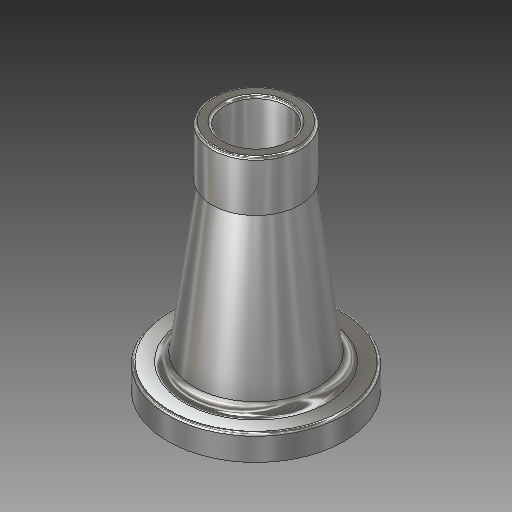
# Autodesk Inventor part: Body
Saved by Autodesk Inventor 2018 (Build 220112000, 112)
## iProperties
Created: 2019-08-24
Part Number: Body
Material: Generic
Document SubType Name: Modeling
Designer: HP
Density: 1 g/cm^3
Appearance: Chrome - Polished
Author: HP
Autodesk Inventor part; units mm, degrees
ref_plane "YZ Plane" through (0, 0, 0) normal (1, 0, 0) x (0, 1, 0)
ref_plane "XZ Plane" through (0, 0, 0) normal (0, 1, 0) x (-1, 0, 0)
ref_plane "XY Plane" through (0, 0, 0) normal (0, 0, 1) x (1, 0, 0)
sketch "Sketch1" plane through (0, 0, 0) normal (0, 0, 1) x (1, 0, 0)
  line L0 (70, 0) -> (50, 0)
  line L1 (50, 0) -> (50, 3)
  line L2 (70, 0) -> (70, 20)
  line L3 (70, 20) -> (50, 20)
  line L4 (25, 185) -> (35, 185)
  line L5 (35, 185) -> (35, 145)
  line L6 (35, 145) -> (33, 145)
  line L7 (33, 145) -> (50, 20)
  line L8 (25, 95.3406) -> (37.5583, 3)
  line L9 (50, 3) -> (37.5583, 3)
  line L10 (25, 185) -> (25, 95.3406)
  line L11 (0, -37) -> (0, 222) projected
  point P0 (0, 0)
  dimension "d0" = 20
  dimension "d1" = 3
  dimension "d2" = 20
  dimension "d3" = 20
  dimension "d4" = 10
  dimension "d5" = 40
  dimension "d6" = 2
  constraints: 22 end point, 4 horizontal, 3 perpendicular, 2 vertical, 1 parallel
  measures "d0" distance of L0.start L0.end
  measures "d1" distance of L0.end L1.end
  measures "d2" distance of L0.start L2.end
  measures "d3" distance of L2.end L3.end
  measures "d4" distance of L4.start L4.end
  measures "d5" distance of L4.end L5.end
  measures "d6" distance of L5.end L6.end
revolve "Revolution1" add sketch "Sketch1" angle 360 about axis through (0, -10, 0) along (0, 1, 0)
fillet "Fillet1" radius 2 1 edges at (-70, 20, 0)
fillet "Fillet2" radius 2 1 edges at (-35, 185, 0)
fillet "Fillet3" radius 2 1 edges at (-25, 185, 0)
fillet "Fillet4" radius 8 1 edges at (-50, 20, 0)
body "Solid1"
